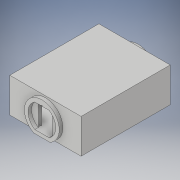
# Autodesk Inventor part: main room
Saved by Autodesk Inventor 2017 (Build 210142000, 142)
## iProperties
Created: 2018-03-03
Part Number: main room
Material: Generic
Document SubType Name: Modeling
Designer: Braxton
Density: 1 g/cm^3
Appearance: Default
Author: Braxton
Autodesk Inventor part; units mm, degrees
ref_plane "YZ Plane" through (0, 0, 0) normal (1, 0, 0) x (0, 1, 0)
sketch "Sketch1" plane through (0, 0, 0) normal (0, 1, 0) x (-1, 0, 0)
  line L0 (0, 0) -> (508, 0)
  line L1 (508, 0) -> (508, -635)
  line L2 (508, -635) -> (0, -635)
  line L3 (0, -635) -> (0, 0)
  dimension "d0" = 508
  dimension "d1" = 635
  constraints: 8 end point, 2 parallel, 1 horizontal, 1 perpendicular
  measures "d0" distance of L1.end L2.end
  measures "d1" distance of L0.end L1.end
extrude "floor" add sketch "Sketch1" along normal blind 25.4
sketch "Sketch4" plane through (0, 25.4, 0) normal (0, 1, 0) x (1, 0, 0)
  line L0 (-508, 0) -> (0, 0) projected
  line L1 (0, 0) -> (0, 635) projected
  line L2 (0, 0) -> (0, 635)
  line L3 (0, 635) -> (-508, 635) projected
  line L4 (0, 635) -> (-508, 635)
  line L5 (-508, 635) -> (-508, 0)
  line L6 (-508, 0) -> (0, 0)
  line L7 (-25.4, 25.4) -> (-482.6, 25.4)
  line L8 (-482.6, 25.4) -> (-482.6, 609.6)
  line L9 (-482.6, 609.6) -> (-25.4, 609.6)
  line L10 (-25.4, 609.6) -> (-25.4, 25.4)
  dimension "d11" = 25.4
  dimension "d12" = 25.4
  dimension "d13" = 25.4
  dimension "d14" = 25.4
  constraints: 16 end point, 4 perpendicular, 3 equal length, 1 horizontal
  measures "d11" distance between parallel lines of L0 L7
  measures "d12" distance between parallel lines of L1 L10
  measures "d13" distance between parallel lines of L3 L9
  measures "d14" distance between parallel lines of L5 L8
extrude "walls" add sketch "Sketch4" along normal blind 220.1333
sketch "Sketch5" plane through (-508, 0, 0) normal (0, 0, 1) x (1, 0, 0)
  line L0 (25.4, 25.4) -> (482.6, 25.4) projected
  line L1 (254, 25.4) -> (304.8, 25.4)
  line L2 (304.8, 25.4) -> (304.8, 194.7333)
  line L3 (304.8, 194.7333) -> (254, 194.7333)
  line L4 (254, 194.7333) -> (254, 25.4)
  line L5 (254, 25.4) -> (203.2, 25.4)
  line L6 (203.2, 25.4) -> (203.2, 194.7333)
  line L7 (203.2, 194.7333) -> (254, 194.7333)
  point P0 (508, 0)
  dimension "d17" = 50.8
  dimension "d18" = 169.3333
  constraints: 14 end point, 2 perpendicular, 2 symmetric about line, 1 horizontal, 1 midpoint, 1 point on line
  measures "d17" distance of L1.start L1.end
  measures "d18" distance of L1.end L2.end
extrude "doorframe" cut sketch "Sketch5" against normal blind 220.1333
sketch "Sketch7" plane through (0, 245.5333, 0) normal (0, 1, 0) x (1, 0, 0)
  line L0 (-482.6, 25.4) -> (-482.6, 609.6) projected
  line L1 (-25.4, 25.4) -> (-25.4, 609.6) projected
  line L2 (-482.6, 609.6) -> (-25.4, 609.6)
  line L3 (-25.4, 609.6) -> (-25.4, 25.4)
  line L4 (-25.4, 25.4) -> (-482.6, 25.4)
  line L5 (-482.6, 25.4) -> (-482.6, 609.6)
  point P0 (0, 0)
  constraints: 8 end point, 2 parallel, 1 horizontal, 1 perpendicular
extrude "ceiling" add sketch "Sketch7" against normal blind 25.4
sketch "Sketch8" plane through (-304.8, 25.4, 0) normal (1, 0, 0) x (0, 0, -1)
  line L0 (12.7, 169.3333) -> (19.05, 169.3333)
  line L1 (19.05, 169.3333) -> (19.05, 0)
  line L2 (19.05, 0) -> (6.35, 0)
  line L3 (6.35, 0) -> (6.35, 169.3333)
  line L4 (12.7, 169.3333) -> (6.35, 169.3333)
  point P0 (0, -25.4)
  point P1 (0, 169.3333)
  point P2 (25.4, 169.3333)
  point P3 (0, 0)
  point P4 (25.4, 0)
  dimension "d24" = 6.35
  dimension "d25" = 12.7
  dimension "d28" = 169.3333
  constraints: 10 end point, 1 horizontal
  measures "d24" distance of L0.start L0.end
  measures "d25" distance of L1.end L2.end
  measures "d28" distance between parallel lines of L2 L0
extrude "left door slot" cut sketch "Sketch8" against normal blind 50.8
ref_plane "mirror door slot" through (-254, 25.4, 0) normal (1, 0, 0) x (0, 0, -1)
mirror "right door slot" about plane through (-254, 25.4, 0) normal (1, 0, 0) of "left door slot"
sketch "Sketch10" plane through (-508, 0, 0) normal (0, 0, 1) x (1, 0, 0)
  line L0 (203.2, 25.4) -> (304.8, 25.4)
  arc A0 (311.4059, 0) -> (196.5941, 0) centre (254, 110.0667) ccw
  arc A1 (203.2, 194.7333) -> (203.2, 25.4) centre (254, 110.0667) ccw
  arc A2 (304.8, 25.4) -> (304.8, 194.7333) centre (254, 110.0667) ccw
  line L1 (203.2, 194.7333) -> (304.8, 194.7333) projected
  line L2 (203.2, 194.7333) -> (203.2, 25.4) projected
  line L3 (508, 0) -> (0, 0) projected
  line L4 (196.5941, 0) -> (311.4059, 0)
  line L5 (254, 194.7333) -> (254, 197.9083) construction
  line L6 (246.5917, 197.9083) -> (261.4083, 197.9083)
  line L7 (246.5917, 197.9083) -> (246.5917, 196.3208)
  line L8 (261.4083, 197.9083) -> (261.4083, 196.3208)
  line L9 (261.4083, 194.7333) -> (262.9958, 194.7333) construction
  arc A3 (261.4083, 196.3208) -> (262.9958, 194.7333) centre (262.9958, 196.3208) ccw
  arc A4 (245.0042, 194.7333) -> (246.5917, 196.3208) centre (245.0042, 196.3208) ccw
  line L10 (203.2, 194.7333) -> (245.0042, 194.7333)
  line L11 (262.9958, 194.7333) -> (304.8, 194.7333)
  line L12 (245.0042, 194.7333) -> (262.9958, 194.7333)
  point P0 (203.2, 110.0667)
  dimension "d38" = 101.6
  dimension "d39" = 25.4
  dimension "d42" = 14.8167
  dimension "d43" = 1.5875
  dimension "d44" = 1.5875
  constraints: 20 end point, 10 point on circle, 5 centre point, 4 horizontal, 3 midpoint, 3 point on line, 3 symmetric about line, 2 coincident, 2 parallel, 2 tangent, 1 collinear, 1 vertical, 1 other
  measures "d38" distance of L10.start L11.end
  measures "d39" distance between parallel lines of L0 L3
  measures "d42" distance of L7.start L6.end
  measures "d43" distance from line of L9.end L8
  measures "d44" radius of A3
extrude "corridor connect" add sketch "Sketch10" along normal blind 25.4
sketch "Sketch11" plane through (-508, 245.5333, 0) normal (0, 0, 1) x (1, 0, 0)
  line L0 (247.65, -47.625) -> (254, -47.625)
  line L1 (261.4083, -47.625) -> (246.5917, -47.625)
  line L2 (247.65, -47.625) -> (247.65, -48.8488)
  line L3 (249.8966, -50.8206) -> (254, -50.8206)
  line L4 (254, -50.8206) -> (254, -47.625) construction
  line L5 (247.6515, -50.8) -> (250.8265, -47.625) construction
  arc A0 (250.8264, -50.8206) -> (247.65, -47.625) centre (247.6515, -50.8) ccw construction
  arc A1 (247.65, -48.8488) -> (249.8966, -50.8206) centre (249.8966, -48.5549) ccw
  line L6 (260.35, -47.625) -> (254, -47.625)
  line L7 (260.35, -47.625) -> (260.35, -48.8488)
  line L8 (258.1034, -50.8206) -> (254, -50.8206)
  line L9 (260.3485, -50.8) -> (257.1735, -47.625) construction
  arc A2 (260.35, -47.625) -> (257.1736, -50.8206) centre (260.3485, -50.8) ccw construction
  arc A3 (258.1034, -50.8206) -> (260.35, -48.8488) centre (258.1034, -48.5549) ccw
  line L10 (246.5917, -47.625) -> (261.4083, -47.625) projected
  point P0 (508, -245.5333)
  dimension "d46" = 6.35
  dimension "d47" = 3.175
  dimension "d48" = 45
  dimension "d49" = 2.2657
  dimension "d50" = 2.2466
  constraints: 20 end point, 10 point on circle, 7 symmetric about line, 6 point on line, 4 centre point, 3 coincident, 2 horizontal, 2 perpendicular, 1 midpoint, 1 tangent, 1 vertical, 2 other
  measures "d46" distance of L4.end L0.start
  measures "d47" distance of L0.start L5.start
  measures "d48" angle of L0 L5
  measures "d49" radius of A1
  measures "d50" horizontal distance of L3.start L2.end
extrude "light" add sketch "Sketch11" along normal up to surface (25.4 mm away) separate body
extrude "into wall light cut" cut sketch "Sketch10" against normal up to surface (6.35 mm away) contours A4 L7 L6 L8 A3 L1 bodies 1
extrude "into wall light join" add sketch "Sketch11" against normal up to surface (6.35 mm away) bodies 1
ref_plane "middle of the room" through (-508, 245.5333, -317.5) normal (0, 0, 1) x (1, 0, 0)
mirror "Mirror connection for starting door" about plane through (-508, 245.5333, -317.5) normal (0, 0, 1) of "doorframe", "corridor connect", "into wall light join", "into wall light cut", "light" bodies 1
equation "\"d12\" = d11"
equation "\"d13\" = d12"
equation "\"d14\" = d13"
equation "\"d43\" = 0.5 * d45"
equation "\"d45\" = 3.175"
body "Solid1"
body "Solid2"
